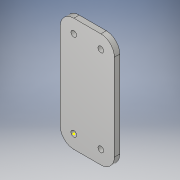
# Autodesk Inventor part: オムニ_固定具4
Saved by Autodesk Inventor 2019.4 (Build 234330000, 330)
## iProperties
Created: 2021-12-04
Part Number: オムニ_固定具4
Material: アルミニウム 6061
Document SubType Name: Modeling
Designer: 堀川皓史
Density: 2.7 g/cm^3
Appearance: アルミニウム - フラット
Author: 堀川皓史
Autodesk Inventor part; units mm, degrees
ref_plane "YZ Plane" through (0, 0, 0) normal (1, 0, 0) x (0, 1, 0)
ref_plane "XZ Plane" through (0, 0, 0) normal (0, 1, 0) x (-1, 0, 0)
ref_plane "XY Plane" through (0, 0, 0) normal (0, 0, 1) x (1, 0, 0)
sketch "スケッチ1" plane through (0, 0, 0) normal (0, 0, 1) x (1, 0, 0)
  circle A0 centre (0, 0) radius 1.6
  circle A1 centre (15, 0) radius 1.6
  circle A2 centre (0, 48) radius 1.6
  circle A3 centre (15, 48) radius 1.6
  line L0 (-7.5, -7.5) -> (22.5, -7.5)
  line L1 (22.5, -7.5) -> (22.5, 55.5)
  line L2 (22.5, 55.5) -> (-7.5, 55.5)
  line L3 (-7.5, 55.5) -> (-7.5, -7.5)
  dimension "d0" = 3.2
  dimension "d1" = 3.2
  dimension "d2" = 3.2
  dimension "d3" = 3.2
  dimension "d4" = 15
  dimension "d5" = 48
  dimension "d6" = 7.5
  dimension "d7" = 7.5
  dimension "d8" = 7.5
  dimension "d9" = 7.5
  constraints: 8 end point, 4 centre point, 2 horizontal alignment, 2 parallel, 2 vertical alignment, 1 coincident, 1 horizontal, 1 perpendicular
  measures "d0" diameter of A0
  measures "d1" diameter of A1
  measures "d2" diameter of A2
  measures "d3" diameter of A3
  measures "d4" distance of A1.centre point (0, 0)
  measures "d5" distance of A2.centre point (0, 0)
  measures "d6" distance from line of A0.centre L0
  measures "d7" distance from line of A2.centre L2
  measures "d8" distance from line of A0.centre L3
  measures "d9" distance from line of L1 A1.centre
extrude "押し出し1" add sketch "スケッチ1" along normal blind 3
fillet "フィレット1" radius 7.5 4 edges at (-7.5, 55.5, 1.5) (22.5, 55.5, 1.5) (22.5, -7.5, 1.5) (-7.5, -7.5, 1.5)
sketch "スケッチ2" plane through (0, 0, 3) normal (0, 0, 1) x (1, 0, 0)
  point P0 (0, 0)
